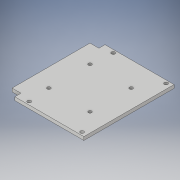
# Autodesk Inventor part: 000,105 - Дно переднего сегмента
Saved by Autodesk Inventor 2019 (Build 230136000, 136)
## iProperties
Created: 2020-06-06
Part Number: 000,105 - Дно переднего сегмента
Material: Типовые
Document SubType Name: Modeling
Designer: Петров Иван
Density: 1 g/cm^3
Appearance: По умолчанию
Author: Петров Иван
Autodesk Inventor part; units mm, degrees
ref_plane "YZ Plane" through (0, 0, 0) normal (1, 0, 0) x (0, 1, 0)
ref_plane "XZ Plane" through (0, 0, 0) normal (0, 1, 0) x (-1, 0, 0)
ref_plane "XY Plane" through (0, 0, 0) normal (0, 0, 1) x (1, 0, 0)
sketch "Эскиз1" plane through (0, 0, 0) normal (0, 1, 0) x (-1, 0, 0)
  circle A0 centre (16.875, 37.75) radius 1.6
  circle A1 centre (-30.625, 37.75) radius 1.6
  line L0 (-35, 40.5) -> (27, 40.5)
  line L1 (-35, 35) -> (-35, 40.5)
  line L2 (27, 35) -> (-35, 35)
  line L3 (27, 40.5) -> (27, 35)
  circle A2 centre (16.875, -37.75) radius 1.6
  circle A3 centre (-30.625, -37.75) radius 1.6
  line L4 (-35, -40.5) -> (27, -40.5)
  line L5 (27, -40.5) -> (27, -35)
  line L6 (-35, -35) -> (27, -35)
  line L7 (-35, -35) -> (-35, -40.5)
  line L8 (35, -35) -> (27, -35)
  line L9 (35, -35) -> (35, -20)
  line L10 (35, -20) -> (35, 20)
  line L11 (35, 20) -> (35, 35)
  line L12 (35, 35) -> (27, 35)
  line L13 (-35, 20) -> (-35, -20)
  line L14 (-35, 35) -> (-35, 20)
  line L15 (-35, -20) -> (-35, -35)
  point P0 (0, 0)
  point P1 (0, 0)
  constraints: 32 end point, 4 centre point
extrude "Выдавливание1" add sketch "Эскиз1" along normal blind 3
sketch "Эскиз2" plane through (0, 3, 0) normal (0, 1, 0) x (1, 0, 0)
  line L0 (-21.5, -21.875) -> (-21.5, 21.875)
  line L1 (21.5, -21.875) -> (-21.5, -21.875)
  line L2 (21.5, 21.875) -> (21.5, -21.875)
  line L3 (-21.5, 21.875) -> (21.5, 21.875)
  circle A0 centre (18.5, -18.5) radius 1.5
  circle A1 centre (-18.5, -18.5) radius 1.5
  circle A2 centre (-18.5, 18.5) radius 1.5
  circle A3 centre (18.5, 18.5) radius 1.5
  point P0 (0, 0)
  point P1 (0, 0)
  constraints: 8 end point, 4 centre point
extrude "Выдавливание2" cut sketch "Эскиз2" against normal blind 10 contours A0 | A1 | A2 | A3
